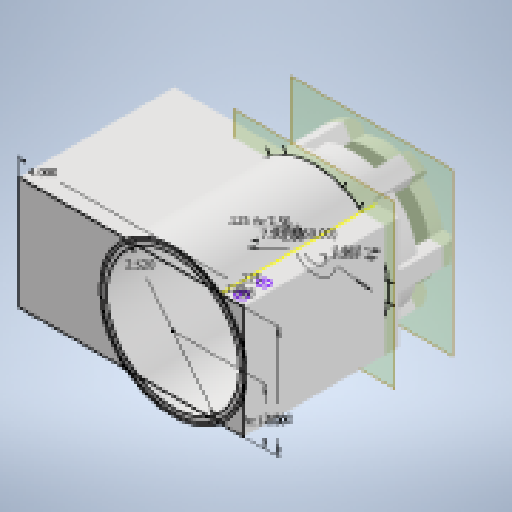
# Autodesk Inventor part: Part142
Saved by Autodesk Inventor 2023 (Build 270158000, 158)
## iProperties
Created: 2023-03-28
Part Number: Part142
Material: Generic
Document SubType Name: Modeling
Designer: Gabriel - T3 CAD
Density: 1 g/cm^3
Appearance: Default
Author: Gabriel - T3 CAD
Autodesk Inventor part; units mm, degrees
ref_plane "YZ Plane" through (0, 0, 0) normal (1, 0, 0) x (0, 1, 0)
ref_plane "XZ Plane" through (0, 0, 0) normal (0, 1, 0) x (-1, 0, 0)
ref_plane "XY Plane" through (0, 0, 0) normal (0, 0, 1) x (1, 0, 0)
sketch "Sketch1" plane through (0, 0, 0) normal (0, 0, 1) x (1, 0, 0)
  circle A0 centre (0, 0) radius 31
  circle A1 centre (0, 0) radius 34.175
  dimension "d0" = 62
  dimension "d1" = 68.35
  constraints: 3 coincident, 2 centre point
  measures "d0" diameter of A0
  measures "d1" diameter of A1
extrude "Extrusion1" add sketch "Sketch1" along normal blind 6.35
ref_plane "Work Plane1" through (0, 0, -83.5) normal (0, 0, -1) x (-1, 0, 0)
sketch "Sketch2" plane through (0, 0, -83.5) normal (0, 0, -1) x (-1, 0, 0)
  circle A0 centre (0, 0) radius 30
  circle A1 centre (0, 0) radius 33.175
  circle A2 centre (0, 0) radius 23
  circle A3 centre (0, 0) radius 26.175
  dimension "d5" = 60
  dimension "d6" = 66.35
  dimension "d28" = 46
  dimension "d29" = 52.35
  constraints: 9 coincident, 4 centre point
  measures "d5" diameter of A0
  measures "d6" diameter of A1
  measures "d28" diameter of A2
  measures "d29" diameter of A3
ref_plane "Work Plane2" through (0, 0, -57.65) normal (0, 0, -1) x (-1, 0, 0)
sketch "Sketch3" plane through (0, 0, -57.65) normal (0, 0, -1) x (-1, 0, 0)
  circle A0 centre (0, 0) radius 34.175
  circle A1 centre (0, 0) radius 31
  circle A2 centre (0, 0) radius 24
  circle A3 centre (0, 0) radius 27.175
  line L0 (0, 0) -> (34.175, 0)
  line L1 (0, 0) -> (34.175, 0) construction
  line L2 (0, 0) -> (33.8826, 4.4607)
  line L3 (0, 0) -> (33.8826, -4.4607)
  line L4 (33.8826, 4.4607) -> (33.8826, -4.4607)
  line L5 (33.8826, -4.4607) -> (0, -4.4607)
  line L6 (0, -4.4607) -> (0, 4.4607)
  line L7 (0, 4.4607) -> (33.8826, 4.4607)
  line L8 (33.8826, 4.4607) -> (33.8826, -4.4607)
  line L9 (33.8826, -4.4607) -> (37.0576, -4.4607)
  line L10 (37.0576, -4.4607) -> (37.0576, 4.4607)
  line L11 (37.0576, 4.4607) -> (33.8826, 4.4607)
  line L12 (-3.8631, 2.2304) -> (13.0782, 31.5736)
  line L13 (20.8044, 27.1129) -> (3.8631, -2.2304)
  line L14 (20.8044, 27.1129) -> (22.3919, 29.8625)
  line L15 (14.6657, 34.3232) -> (13.0782, 31.5736)
  line L16 (-3.8631, -2.2304) -> (-20.8044, 27.1129)
  line L17 (-13.0782, 31.5736) -> (3.8631, 2.2304)
  line L18 (-13.0782, 31.5736) -> (-14.6657, 34.3232)
  line L19 (-22.3919, 29.8625) -> (-20.8044, 27.1129)
  line L20 (0, -4.4607) -> (-33.8826, -4.4607)
  line L21 (-33.8826, 4.4607) -> (0, 4.4607)
  line L22 (-33.8826, 4.4607) -> (-37.0576, 4.4607)
  line L23 (-37.0576, -4.4607) -> (-33.8826, -4.4607)
  line L24 (3.8631, -2.2304) -> (-13.0782, -31.5736)
  line L25 (-20.8044, -27.1129) -> (-3.8631, 2.2304)
  line L26 (-20.8044, -27.1129) -> (-22.3919, -29.8625)
  line L27 (-14.6657, -34.3232) -> (-13.0782, -31.5736)
  line L28 (3.8631, 2.2304) -> (20.8044, -27.1129)
  line L29 (13.0782, -31.5736) -> (-3.8631, -2.2304)
  line L30 (13.0782, -31.5736) -> (14.6657, -34.3232)
  line L31 (22.3919, -29.8625) -> (20.8044, -27.1129)
  line L32 (-34.175, 6.35) -> (0, 6.35)
  line L33 (0, 6.35) -> (0, -6.35)
  line L34 (0, -6.35) -> (-34.175, -6.35)
  line L35 (-34.175, -6.35) -> (-34.175, 6.35)
  line L36 (-9.525, 34.175) -> (9.525, 34.175)
  line L37 (9.525, 34.175) -> (9.525, 0)
  line L38 (9.525, 0) -> (-9.525, 0)
  line L39 (-9.525, 0) -> (-9.525, 34.175)
  point P0 (-26.8064, 4.4607)
  point P1 (-33.8826, 4.4607)
  point P2 (-33.8826, -4.4607)
  point P3 (-26.8064, -4.4607)
  point P4 (-17.2663, -20.9846)
  point P5 (-20.8044, -27.1129)
  point P6 (-13.0782, -31.5736)
  point P7 (-9.5401, -25.4454)
  point P8 (9.5401, -25.4454)
  point P9 (20.8044, -27.1129)
  point P10 (17.2663, -20.9846)
  point P11 (26.8064, -4.4607)
  point P12 (26.8064, 4.4607)
  point P13 (17.2663, 20.9846)
  point P14 (20.8044, 27.1129)
  point P15 (13.0782, 31.5736)
  point P16 (9.5401, 25.4454)
  point P17 (-13.0782, 31.5736)
  point P18 (-20.8044, 27.1129)
  point P19 (-17.2663, 20.9846)
  point P20 (-9.5401, 25.4454)
  point P21 (-34.175, 0)
  point P22 (0, 0)
  point P23 (0, 0)
  point P24 (-7.9278, 22.6528)
  point P25 (-9.525, 25.4192)
  point P26 (-9.525, 29.5004)
  point P27 (9.525, 29.5004)
  point P28 (9.525, 25.4192)
  point P29 (7.9278, 22.6528)
  point P30 (-9.525, 22.0289)
  point P31 (9.525, 22.0289)
  dimension "d8" = 68.35
  dimension "d9" = 62
  dimension "d10" = 48
  dimension "d11" = 54.35
  dimension "d12" = 0
  dimension "d13" = 7.5
  dimension "d14" = 7.5
  dimension "d15" = 3.175
  dimension "d18" = 360
  dimension "d70" = 12.7
  dimension "d71" = 19.05
  dimension "d72" = 9.525
  constraints: 80 end point, 10 coincident, 8 parallel, 6 midpoint, 4 centre point, 4 perpendicular, 3 horizontal, 3 point on circle, 2 tangent, 1 collinear, 1 point on line, 61 other
  measures "d8" diameter of A0
  measures "d9" diameter of A1
  measures "d10" diameter of A2
  measures "d11" diameter of A3
  measures "d12" distance between parallel lines of L0 L1
  measures "d13" angle of L0 L3
  measures "d14" angle of L0 L2
  measures "d15" distance of L9.end L3.end
  measures "d70" distance of L34.end L32.start
  measures "d71" distance of L36.start L36.end
  measures "d72" distance from line of point (0, 0) L39
extrude "Extrusion2" add sketch "Sketch3" against normal up to surface (57.65 mm away) contours L0 L4 A0 | A0 L4 L0 | L7 A1 L13 A0 | L4 L0 A1 L2 | L2 A1 L7 | L5 A1 L3 | L3 A1 L0 L4 | A0 L28 A1 L5 | L13 A1 L12 A0 | A0 L29 A1 L28 | L12 A1 L37 A0 | A0 L24 A1 L29 | L37 A1 L39 A0 | A0 L25 A1 L24 | A0 L34 A1 L25 | L39 A1 L17 A0 | A0 L20 A1 L34 | L17 A1 L16 A0 | A0 L21 A1 L20 | L16 A1 L32 A0 | L32 A1 L21 A0
extrude "Extrusion3" add sketch "Sketch3" along normal blind 17 contours L2 A3 L7 A1 | A1 L0 A3 L2 | L7 A3 L13 A1 | L3 A3 L0 A1 | A1 L5 A3 L3 | A1 L28 A3 L5 | L13 A3 L12 A1 | L2 A2 L7 A3 | A3 L0 A2 L2 | L7 A2 L13 A3 | A1 L29 A3 L28 | L3 A2 L0 A3 | A3 L5 A2 L3 | A3 L28 A2 L5 | L12 A3 L37 A1 | L13 A2 L37 L12 A3 | A1 L24 A3 L29 | A3 L29 A2 L28 | L12 L37 A3 | A1 L25 A3 L24 | A3 L24 A2 L29 | L39 A3 L17 A1 | A1 L34 A3 L25 | A3 L25 A2 L24 | L17 A3 L16 A1 | L39 L17 A3 | A1 L20 A3 L34 | A3 L34 A2 L25 | L16 A3 L32 A1 | L17 L39 A2 L16 A3 | A1 L21 A3 L20 | A3 L20 A2 L34 | L32 A3 L21 A1 | L16 A2 L32 A3 | A3 L21 A2 L20 | L32 A2 L21 A3
extrude "Extrusion5" add sketch "Sketch3" along normal blind 6.35 contours L0 L4 A0 | A0 L4 L0 | L7 A1 L13 A0 | L4 L0 A1 L2 | L2 A1 L7 | L5 A1 L3 | L3 A1 L0 L4 | A0 L28 A1 L5 | L13 A1 L12 A0 | A0 L29 A1 L28 | L12 A1 L37 A0 | A0 L24 A1 L29 | L37 A1 L39 A0 | A0 L25 A1 L24 | A0 L34 A1 L25 | L39 A1 L17 A0 | A0 L20 A1 L34 | L17 A1 L16 A0 | A0 L21 A1 L20 | L16 A1 L32 A0 | L32 A1 L21 A0
sketch "Sketch4" plane through (0, 0, 6.35) normal (0, 0, 1) x (1, 0, 0)
  circle A0 centre (0, 0) radius 32
  line L0 (32, 25.4) -> (32, -25.4)
  line L1 (32, -25.4) -> (-69.6, -25.4)
  line L2 (-69.6, -25.4) -> (-69.6, 25.4)
  line L3 (-69.6, 25.4) -> (32, 25.4)
  circle A1 centre (0, 0) radius 31
  circle A2 centre (0, 0) radius 31 projected
  circle A3 centre (0, 0) radius 34.175
  circle A4 centre (0, 0) radius 34.175 projected
  point P0 (22.8642, 25.4)
  point P1 (-22.8642, 25.4)
  point P2 (-22.8642, -25.4)
  point P3 (22.8642, -25.4)
  point P4 (32, 11.9971)
  point P5 (32, -11.9971)
  dimension "d41" = 64
  dimension "d42" = 25.4
  dimension "d43" = 50.8
  dimension "d44" = 101.6
  constraints: 8 end point, 3 centre point, 3 coincident, 2 concentric, 2 parallel, 1 horizontal, 1 perpendicular, 1 tangent
  measures "d41" diameter of A0
  measures "d42" distance from line of L1 point (0, 0)
  measures "d43" distance of L0.start L0.end
  measures "d44" distance of L2.end L0.start
extrude "Extrusion7" add sketch "Sketch4" against normal up to surface (70.35 mm away) contours A0 L1 A1 L3 | L0 A3 L1 A0 | A0 L3 A3 L0 | L3 A1 A0 | A0 L3 A3 | L1 A3 A0 | A0 L1 A1 | A3 L3 L0 | L0 L1 A3 | L3 A1 L1 A0 | A0 L1 A3 L3 | A3 L1 L2 L3
extrude "Extrusion8" cut sketch "Sketch4" against normal through all contours L0 A3
sketch "Sketch8" plane through (-69.6, 25.4, 6.35) normal (0, 1, 0) x (1, 0, 0)
  circle A0 centre (12.7, 12.7) radius 2.5797
  line L0 (0, 0) -> (0, 70.35) projected
  line L1 (0, 0) -> (12.7, 0)
  line L2 (0, 0) -> (12.7, 0) construction
  line L3 (0, 0) -> (0, 12.7)
  line L4 (0, 0) -> (12.7, 0) construction
  circle A1 centre (25.4, 12.7) radius 2.5797
  circle A2 centre (12.7, 57.65) radius 2.5797
  circle A3 centre (25.4, 57.65) radius 2.5797
  line L5 (46.7358, 0) -> (0, 0) projected
  line L6 (46.7358, 70.35) -> (0, 70.35) projected
  point P0 (69.6, 6.35)
  dimension "d73" = 12.7
  dimension "d74" = 0
  dimension "d75" = 12.7
  dimension "d76" = 90
  dimension "d79" = 12.7
  dimension "d82" = 44.95
  dimension "d85" = 5.1594
  dimension "d86" = 12.7
  dimension "d87" = 12.7
  dimension "d88" = 12.7
  constraints: 8 end point, 4 centre point, 3 horizontal, 2 equal length, 1 perpendicular, 1 vertical, 6 other
  measures "d73" distance of L0.start L1.end
  measures "d74" distance between parallel lines of L1 L2
  measures "d75" distance of L0.start L3.end
  measures "d76" angle of L4 L3
  measures "d79" distance of A0.centre A1.centre
  measures "d82" distance of A0.centre A2.centre
  measures "d85" diameter of A0
  measures "d86" distance from line of L0 A0.centre
  measures "d87" distance from line of A0.centre L5
  measures "d88" distance from line of L6 A2.centre
extrude "Extrusion11" cut sketch "Sketch8" against normal through all
equation "\"d14\" = d13"
equation "\"d72\" = 0.5 * d71"
equation "\"d42\" = 0.5 * d43"
body "Solid1"
